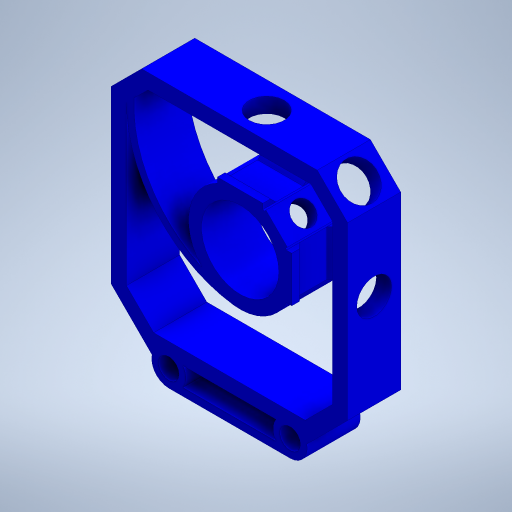
# Autodesk Inventor part: Laser Holder (Blue Laser)
Saved by Autodesk Inventor 2023.1 (Build 271208000, 208)
## iProperties
Created: 2022-07-25
Part Number: Laser Holder (Blue Laser)
Material: Generic
Document SubType Name: Modeling
Designer: xSibe
Density: 1 g/cm^3
Appearance: Plastic Blue
Author: xSibe
Autodesk Inventor part; units mm, degrees
ref_plane "YZ Plane" through (0, 0, 0) normal (1, 0, 0) x (0, 1, 0)
ref_plane "XZ Plane" through (0, 0, 0) normal (0, 1, 0) x (-1, 0, 0)
sketch "Sketch1" plane through (0, 0, 0) normal (0, 0, 1) x (1, 0, 0)
  circle A0 centre (10, 3.85) radius 1.5625 projected
  circle A1 centre (-10, 3.85) radius 1.5625 projected
  line L0 (-16.9, 0) -> (16.9, 0) projected
  line L1 (16.9, 0) -> (16.9, 7.7) projected
  line L2 (-16.9, 7.7) -> (16.9, 7.7) projected
  line L3 (-16.9, 0) -> (-16.9, 7.7) projected
  circle A2 centre (-10, 3.85) radius 2.8125
  circle A3 centre (10, 3.85) radius 2.8125
  line L4 (-10, 6.6625) -> (10, 6.6625)
  line L5 (10, 1.0375) -> (-10, 1.0375)
  line L6 (-10, 2.2875) -> (10, 2.2875)
  line L7 (-10, 5.4125) -> (10, 5.4125)
  line L8 (-17.05, 7.7) -> (-17.05, 42.1) projected
  line L9 (17.05, 7.7) -> (17.05, 42.1) projected
  line L10 (-17.05, 24.9) -> (17.05, 24.9)
  line L11 (0, 24.9) -> (1.7678, 26.6678)
  line L12 (0, 24.9) -> (2.5, 24.9) construction
  circle A4 centre (1.7678, 26.6678) radius 6.375
  circle A5 centre (1.7678, 26.6678) radius 5.7
  circle A6 centre (1.7678, 26.6678) radius 8.5
  line L13 (1.7678, 26.6678) -> (1.7678, 35.1678)
  line L14 (1.7678, 35.1678) -> (1.7678, 34.5428)
  line L15 (-1.9822, 33.9178) -> (5.5178, 33.9178)
  line L16 (5.5178, 33.9178) -> (5.5178, 35.1678)
  line L17 (5.5178, 35.1678) -> (-1.9822, 35.1678)
  line L18 (-1.9822, 35.1678) -> (-1.9822, 33.9178)
  line L19 (-1.9822, 33.9178) -> (5.5178, 35.1678) construction
  line L20 (5.5178, 33.9178) -> (-1.9822, 35.1678) construction
  line L21 (1.7678, 26.6678) -> (7.7782, 32.6782)
  line L22 (7.7782, 32.6782) -> (7.3362, 32.2362)
  line L23 (9.5459, 30.9104) -> (6.0104, 34.4459)
  line L24 (6.0104, 34.4459) -> (5.1265, 33.5621)
  line L25 (5.1265, 33.5621) -> (8.6621, 30.0265)
  line L26 (8.6621, 30.0265) -> (9.5459, 30.9104)
  line L27 (9.5459, 30.9104) -> (5.1265, 33.5621) construction
  line L28 (6.0104, 34.4459) -> (8.6621, 30.0265) construction
  line L29 (9.5459, 30.9104) -> (14.5459, 30.9104) construction
  line L30 (9.0178, 22.9178) -> (9.0178, 30.4178)
  line L31 (9.0178, 30.4178) -> (10.2678, 30.4178)
  line L32 (10.2678, 30.4178) -> (10.2678, 22.9178)
  line L33 (10.2678, 22.9178) -> (9.0178, 22.9178)
  line L34 (1.7678, 35.1678) -> (1.7678, 37.1678)
  line L35 (10.2678, 26.6678) -> (12.2678, 26.6678)
  line L36 (-10.2178, 5.4322) -> (10.2178, 5.4322)
  line L37 (19.4678, 14.6822) -> (19.4678, 39.3678)
  line L38 (14.4678, 44.3678) -> (-14.4678, 44.3678)
  line L39 (-19.4678, 39.3678) -> (-19.4678, 14.6822)
  line L40 (-19.4678, 5.4322) -> (19.4678, 44.3678) construction
  line L41 (19.4678, 5.4322) -> (-19.4678, 44.3678) construction
  line L42 (-10.2178, 5.4322) -> (-19.4678, 14.6822)
  line L43 (10.2178, 5.4322) -> (19.4678, 14.6822)
  line L44 (14.4678, 44.3678) -> (19.4678, 39.3678)
  line L45 (-14.4678, 44.3678) -> (-19.4678, 39.3678)
  line L46 (-15.5033, 46.8678) -> (-21.9678, 40.4033)
  line L47 (-21.9678, 40.4033) -> (-21.9678, 13.6467)
  line L48 (-21.9678, 13.6467) -> (-11.2533, 2.9322)
  line L49 (-11.2533, 2.9322) -> (11.2533, 2.9322)
  line L50 (11.2533, 2.9322) -> (21.9678, 13.6467)
  line L51 (21.9678, 13.6467) -> (21.9678, 40.4033)
  line L52 (21.9678, 40.4033) -> (15.5033, 46.8678)
  line L53 (15.5033, 46.8678) -> (-15.5033, 46.8678)
  line L54 (-13.4322, 41.8678) -> (-16.9678, 38.3322)
  line L55 (-16.9678, 38.3322) -> (-16.9678, 15.7178)
  line L56 (-16.9678, 15.7178) -> (-9.1822, 7.9322)
  line L57 (-9.1822, 7.9322) -> (9.1822, 7.9322)
  line L58 (9.1822, 7.9322) -> (16.9678, 15.7178)
  line L59 (16.9678, 15.7178) -> (16.9678, 38.3322)
  line L60 (16.9678, 38.3322) -> (13.4322, 41.8678)
  line L61 (13.4322, 41.8678) -> (-13.4322, 41.8678)
  line L62 (16.9678, 15.7178) -> (16.9678, 8.6467)
  line L63 (-16.9678, 15.7178) -> (-16.9678, 12.1822)
  line L64 (-19.4678, 14.6822) -> (-19.4678, 11.1467)
  line L65 (19.4678, 14.6822) -> (19.4678, 11.1467)
  arc A7 (-16.9678, 38.3322) -> (0.6633, 18.2398) centre (3.2964, 38.3322) ccw
  arc A8 (-15.6737, 39.6263) -> (-4.5968, 21.0338) centre (3.2964, 38.3322) ccw
  circle A9 centre (-10, 3.85) radius 1.705
  circle A10 centre (10, 3.85) radius 1.707
  point P0 (0, 0)
  point P1 (1.3641, 18.1774)
  point P2 (-3.9462, 20.3748)
  point P3 (-7.6615, 2.2875)
  point P4 (-7.6615, 5.4125)
  point P5 (7.6615, 5.4125)
  point P6 (7.6615, 2.2875)
  point P7 (7.3415, 2.9322)
  point P8 (-7.3415, 2.9322)
  point P9 (-11.1858, 6.4003)
  point P10 (11.1858, 6.4003)
  point P11 (-1.9822, 34.2958)
  point P12 (9.3958, 22.9178)
  point P13 (9.3958, 30.4178)
  point P14 (9.2801, 30.6446)
  point P15 (5.7446, 34.1801)
  point P16 (5.5178, 34.2958)
  point P17 (12.7519, 4.4308)
  point P18 (-12.7519, 4.4308)
  point P19 (5.4822, 33.9178)
  point P20 (-2.842, 34.5428)
  point P21 (9.6428, 22.058)
  point P22 (9.0178, 30.3822)
  point P23 (9.6725, 31.6678)
  point P24 (9.6428, 31.2775)
  point P25 (6.3775, 34.5428)
  point P26 (1.7678, 35.1678)
  point P27 (6.7678, 34.5725)
  point P28 (7.7782, 32.6782)
  point P29 (-17.05, 12.2645)
  point P30 (16.9678, 24.9)
  point P31 (17.05, 12.2645)
  point P32 (-16.9678, 24.9)
  point P33 (16.9678, 12.1822)
  point P34 (10.0819, 24.9)
  point P35 (-6.5464, 24.9)
  point P36 (-17.05, 41.7855)
  point P37 (17.05, 41.7855)
  point P38 (7.6748, 5.4322)
  point P39 (-7.6748, 5.4322)
  point P40 (12.4855, 7.7)
  point P41 (-12.4855, 7.7)
  dimension "d0" = 1.25
  dimension "d1" = 1.25
  dimension "d2" = 2.5
  dimension "d3" = 45
  dimension "d4" = 12.75
  dimension "d5" = 0.675
  dimension "d6" = 2.125
  dimension "d7" = 0.625
  dimension "d8" = 7.5
  dimension "d9" = 1.25
  dimension "d10" = 0.625
  dimension "d11" = 5
  dimension "d12" = 135
  dimension "d13" = 1.25
  dimension "d14" = 2
  dimension "d15" = 2
  dimension "d16" = 38.9355
  dimension "d17" = 38.9355
  dimension "d18" = 9.25
  dimension "d19" = 9.25
  dimension "d20" = 9.25
  dimension "d21" = 9.25
  dimension "d22" = 5
  dimension "d23" = 5
  dimension "d24" = 5
  dimension "d25" = 5
  dimension "d26" = 2.5
  dimension "d46" = 2.5
  dimension "d47" = 1.25
  dimension "d51" = 0.1425
  dimension "d52" = 0.1445
  constraints: 120 end point, 18 point on circle, 16 point on line, 13 parallel, 10 midpoint, 9 centre point, 9 tangent, 7 perpendicular, 6 horizontal, 4 symmetric about line, 2 equal length, 2 vertical, 1 coincident, 14 other
  measures "d0" radial gap between concentric circles of A1 A2
  measures "d1" radial gap between concentric circles of A0 A3
  measures "d2" distance of L11.start L11.end
  measures "d3" angle of L12 L11
  measures "d4" diameter of A4
  measures "d5" radial gap between concentric circles of A4 A5
  measures "d6" radial gap between concentric circles of A4 A6
  measures "d7" distance of L13.end L14.end
  measures "d8" distance of L17.end L16.end
  measures "d9" distance of L16.end L15.end
  measures "d10" distance of L21.end L22.end
  measures "d11" distance of L23.start L23.end
  measures "d12" angle of L29 L23
  measures "d13" distance of L24.end L23.end
  measures "d14" distance of L13.end L34.end
  measures "d15" distance of L35.start L35.end
  measures "d16" distance of L40.end L41.end
  measures "d17" distance of L41.end L40.start
  measures "d18" distance of L36.start L40.start
  measures "d19" distance of L39.end L40.start
  measures "d20" distance of L36.end L41.start
  measures "d21" distance of L37.start L41.start
  measures "d22" distance of L38.start L40.end
  measures "d23" distance of L37.end L40.end
  measures "d24" distance of L38.end L41.end
  measures "d25" distance of L39.start L41.end
  measures "d26" distance between parallel lines of L38 L53
  measures "d46" distance between parallel lines of L38 L61
  measures "d47" radial gap between concentric circles of A7 A8
  measures "d51" radial gap between concentric circles of A1 A9
  measures "d52" radial gap between concentric circles of A0 A10
extrude "Extrusion1" add sketch "Sketch1" along normal mid plane 8.75 contours A10 L49 A3 L7 | L7 A3 L36 A10 | A10 L43 A3 L50 | L50 A3 L6 A10 | A10 L6 A3 L49 | L7 A2 L36 A3 | L36 A3 L43 A10 | A3 L43 L2 L50 | L36 A2 L4 A3 | L7 A9 L36 A2 | A2 L49 A9 L7 | A3 L5 A2 L6 | A3 L4 A2 L42 L2 L43 | L2 L43 L62 L50 | A2 L6 A9 L49 | L36 A9 L42 A2 | A2 L48 A9 L6 | L62 L43 L9 L50 | L42 A2 L48 L2 | L2 L48 L8 L42 | L62 L59 L10 L9 L43 | L9 L43 L65 L50 | L42 A9 L48 A2 | L42 L8 L10 L55 L63 | L9 L44 L37 L43 | L48 L64 L42 L8 | L42 L39 L45 L8 | L10 L59 L60 L61 L54 L55 L8 L45 L38 L44 L9 | L32 L33 A6 L10 | L10 A6 L32 | A7 L54 A8 L10 | L10 A8 A6 A7 | A6 L33 L30 L10 | L10 L30 L26 L31 A6 | A6 L31 L32 | A6 L10 A4 L30 L33 | L10 A4 L21 L25 L26 L30 | L31 L26 A6 | A6 L18 L15 L13 A4 L10 | L30 L31 L26 | L26 L25 L21 A6 L31 L30 | A6 L23 L26 | L18 L17 A6 | A6 L13 L15 L18 | L21 L25 L24 L15 L16 A6 | A6 L24 L23 | L13 L15 L24 L25 L21 A4 | L17 L16 A6 | A6 L16 L24 L15 L13 | L24 L16 A6 | L16 L15 L24
sketch "Sketch2" plane through (0, 0, 0) normal (0, 0, 1) x (1, 0, 0)
  circle A0 centre (1.7678, 26.6678) radius 6.375 projected
  circle A1 centre (1.7678, 26.6678) radius 5.5
  line L0 (-10, 1.0375) -> (10, 1.0375) projected
  arc A2 (10, 1.0375) -> (12.7519, 4.4308) centre (10, 3.85) ccw projected
  line L1 (12.7519, 4.4308) -> (19.4678, 11.1467) projected
  line L2 (19.4678, 11.1467) -> (19.4678, 39.3678) projected
  line L3 (19.4678, 39.3678) -> (14.4678, 44.3678) projected
  line L4 (14.4678, 44.3678) -> (-14.4678, 44.3678) projected
  line L5 (-14.4678, 44.3678) -> (-19.4678, 39.3678) projected
  line L6 (-19.4678, 39.3678) -> (-19.4678, 11.1467) projected
  line L7 (-19.4678, 11.1467) -> (-12.7519, 4.4308) projected
  arc A3 (-12.7519, 4.4308) -> (-10, 1.0375) centre (-10, 3.85) ccw projected
  line L8 (-7.6615, 5.4125) -> (7.6615, 5.4125) projected
  arc A4 (7.6615, 5.4125) -> (7.6615, 2.2875) centre (10, 3.85) ccw projected
  line L9 (7.6615, 2.2875) -> (-7.6615, 2.2875) projected
  arc A5 (-7.6615, 2.2875) -> (-7.6615, 5.4125) centre (-10, 3.85) ccw projected
  circle A6 centre (1.7678, 26.6678) radius 6.375 projected
  line L10 (5.5178, 35.1678) -> (-1.9822, 35.1678) projected
  line L11 (-1.9822, 35.1678) -> (-1.9822, 34.2958) projected
  arc A7 (-1.9822, 34.2958) -> (-4.5968, 21.0338) centre (1.7678, 26.6678) ccw projected
  arc A8 (-15.6737, 39.6263) -> (-4.5968, 21.0338) centre (3.2964, 38.3322) ccw projected
  line L12 (-15.6737, 39.6263) -> (-13.4322, 41.8678) projected
  line L13 (-13.4322, 41.8678) -> (13.4322, 41.8678) projected
  line L14 (13.4322, 41.8678) -> (16.9678, 38.3322) projected
  line L15 (16.9678, 38.3322) -> (16.9678, 12.1822) projected
  line L16 (16.9678, 12.1822) -> (12.4855, 7.7) projected
  line L17 (12.4855, 7.7) -> (-12.4855, 7.7) projected
  line L18 (-12.4855, 7.7) -> (-16.9678, 12.1822) projected
  line L19 (-16.9678, 12.1822) -> (-16.9678, 38.3322) projected
  arc A9 (-16.9678, 38.3322) -> (0.6633, 18.2398) centre (3.2964, 38.3322) ccw projected
  arc A10 (0.6633, 18.2398) -> (9.3958, 22.9178) centre (1.7678, 26.6678) ccw projected
  line L20 (9.3958, 22.9178) -> (10.2678, 22.9178) projected
  line L21 (10.2678, 22.9178) -> (10.2678, 30.4178) projected
  line L22 (10.2678, 30.4178) -> (9.3958, 30.4178) projected
  arc A11 (9.3958, 30.4178) -> (9.2801, 30.6446) centre (1.7678, 26.6678) ccw projected
  line L23 (9.2801, 30.6446) -> (9.5459, 30.9104) projected
  line L24 (9.5459, 30.9104) -> (6.0104, 34.4459) projected
  line L25 (6.0104, 34.4459) -> (5.7446, 34.1801) projected
  arc A12 (5.7446, 34.1801) -> (5.5178, 34.2958) centre (1.7678, 26.6678) ccw projected
  line L26 (5.5178, 34.2958) -> (5.5178, 35.1678) projected
  circle A13 centre (1.7678, 26.6678) radius 8.5
  point P0 (0, 0)
  point P1 (5.5178, 34.2958)
  point P2 (-1.9822, 34.2958)
  point P3 (0.6633, 18.2398)
  dimension "d30" = 0.875
  constraints: 1 centre point, 1 coincident, 3 other
  measures "d30" radial gap between concentric circles of A0 A1
extrude "Extrusion2" [suppressed]
sketch "Sketch3" plane through (19.4678, 13.6467, -4.375) normal (1, 0, 0) x (0, 0, -1)
  line L0 (0, 9.2711) -> (-8.75, 9.2711) projected
  line L1 (0, 16.7711) -> (0, 9.2711) projected
  line L2 (0, 16.7711) -> (-8.75, 16.7711) projected
  line L3 (-8.75, 9.2711) -> (-8.75, 16.7711) projected
  line L4 (-4.375, 16.7711) -> (-4.375, 9.2711)
  circle A0 centre (-4.375, 13.0211) radius 2.875
  point P0 (-4.375, -13.6467)
  dimension "d33" = 5.75
  constraints: 3 midpoint, 2 end point, 1 centre point
  measures "d33" diameter of A0
extrude "Extrusion3" cut sketch "Sketch3" against normal up to surface (2.5 mm away) contours A0 L4 | L4 A0
sketch "Sketch4" plane through (9.3958, 30.4178, -4.375) normal (0, 1, 0) x (1, 0, 0)
  line L0 (0.8719, 0) -> (0.8719, -8.75) projected
  line L1 (0, 0) -> (0.8719, 0) projected
  line L2 (0.8719, -8.75) -> (0, -8.75) projected
  line L3 (0.8719, -8.75) -> (0, -8.75)
  line L4 (0, -8.75) -> (0, -7.5)
  line L5 (0, -7.5) -> (0.8719, -7.5)
  line L6 (0.8719, -7.5) -> (0.8719, -8.75)
  line L7 (0.8719, -7.5) -> (0, -6.6281)
  line L8 (0.8719, -7.5) -> (2.105, -7.5) construction
  line L9 (0, -4.375) -> (0.8719, -4.375)
  line L10 (0.8719, -1.25) -> (0, -2.1219)
  line L11 (0, 0) -> (0, -8.75) projected
  point P0 (-9.3958, -4.375)
  point P1 (0.8719, -1.25)
  point P2 (0.8719, -7.5)
  point P3 (0, -6.6938)
  point P4 (0, -2.1219)
  point P5 (0.8719, -7.5)
  dimension "d36" = 1.25
  dimension "d37" = 135
  constraints: 16 end point, 2 horizontal, 2 midpoint, 2 parallel, 2 point on line, 2 symmetric about line, 1 equal length, 1 perpendicular
  measures "d36" distance of L3.end L4.end
  measures "d37" angle of L8 L7
extrude "Extrusion4" cut sketch "Sketch4" against normal up to surface (7.5 mm away) contours L0 L9 L11 L10 | L0 L7 L11 L9
ref_plane "Work Plane1" through (10.2678, 35.1678, 4.375) normal (0.7071068, -0.7071068, 0) x (0, 0, -1)
mirror "Mirror1" about plane through (10.2678, 35.1678, 4.375) normal (0.7071068, -0.7071068, 0) of "Extrusion3", "Extrusion4"
sketch "Sketch5" plane through (20.2, 38.6355, 4.375) normal (0.7071068, 0.7071068, 0) x (0.7071068, -0.7071068, 0)
  circle A0 centre (-4.5711, 4.375) radius 1.875
  line L0 (-8.1066, 4.375) -> (-1.0355, 4.375)
  circle A1 centre (-4.5711, 4.375) radius 3
  line L1 (-8.1066, 8.75) -> (-8.1066, 0) projected
  line L2 (-1.0355, 0) -> (-8.1066, 0) projected
  line L3 (-1.0355, 8.75) -> (-1.0355, 0) projected
  line L4 (-8.1066, 8.75) -> (-1.0355, 8.75) projected
  point P0 (13.0359, 4.375)
  dimension "d40" = 3.75
  dimension "d41" = 6
  constraints: 3 midpoint, 2 centre point, 2 end point, 1 coincident
  measures "d40" diameter of A0
  measures "d41" diameter of A1
extrude "Extrusion5" cut sketch "Sketch5" against normal blind 5 contours L0 A0 | L0 A1 A0 | A0 L0 A1 | A0 L0
extrude "Extrusion6" cut sketch "Sketch5" against normal up to next from surface at -12.996 contours L0 A0 | A0 L0
pattern_linear "Rectangular Pattern1" [suppressed]
equation "\"d19\" = d18"
equation "\"d20\" = d18"
equation "\"d21\" = d20"
equation "\"d23\" = d22"
equation "\"d24\" = d22"
equation "\"d25\" = d24"
body "Solid1"
